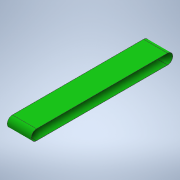
# Autodesk Inventor part: Băng tải
Saved by Autodesk Inventor 2020 (Build 240168000, 168)
## iProperties
Created: 2022-12-09
Part Number: Băng tải
Material: Generic
Document SubType Name: Modeling
Designer: ADMIN
Density: 1 g/cm^3
Appearance: Default
Author: ADMIN
Autodesk Inventor part; units mm, degrees
ref_plane "YZ Plane" through (0, 0, 0) normal (1, 0, 0) x (0, 1, 0)
ref_plane "XZ Plane" through (0, 0, 0) normal (0, 1, 0) x (-1, 0, 0)
ref_plane "XY Plane" through (0, 0, 0) normal (0, 0, 1) x (1, 0, 0)
sketch "Sketch1" plane through (0, 0, 0) normal (1, 0, 0) x (0, 1, 0)
  arc A0 (19.5, 0) -> (-19.5, 0) centre (0, 0) ccw
  arc A1 (-19.5, -490) -> (19.5, -490) centre (0, -490) ccw
  line L0 (19.5, 0) -> (19.5, -490)
  line L1 (-19.5, 0) -> (-19.5, -490)
  dimension "d0" = 39
  dimension "d1" = 39
  dimension "d2" = 490
  constraints: 4 end point, 4 point on circle, 2 centre point, 2 tangent, 1 coincident, 1 vertical
  measures "d0" diameter of A0
  measures "d1" diameter of A1
  measures "d2" distance of L0.start L0.end
extrude "Extrusion1" add sketch "Sketch1" along normal blind 90
sketch "Sketch2" plane through (0, 0, 0) normal (-1, 0, 0) x (0, 0, 1)
  arc A0 (0, -19) -> (0, 19) centre (0, 0) ccw
  arc A1 (-490, 19.5) -> (-490, -19.5) centre (-490, 0) ccw projected
  arc A2 (-490, 19) -> (-490, -19) centre (-490, 0) ccw
  line L0 (-490, 19) -> (0, 19)
  line L1 (0, -19) -> (-490, -19)
  dimension "d5" = 38
  dimension "d6" = 38
  constraints: 4 end point, 4 point on circle, 3 tangent, 2 centre point, 2 coincident, 1 parallel
  measures "d5" diameter of A0
  measures "d6" diameter of A2
extrude "Extrusion2" cut sketch "Sketch2" against normal through all
body "Solid1"
